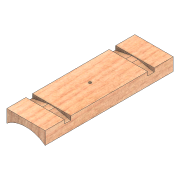
# Autodesk Inventor part: legno 2
Saved by Autodesk Inventor 2022 (Build 260153000, 153)
## iProperties
Created: 2025-08-09
Part Number: legno 2
Material: Wood (Birch)
Document SubType Name: Modeling
Designer: sacchie
Density: 0.55 g/cm^3
Appearance: Birch - Natural Polished
Author: sacchie
Autodesk Inventor part; units mm, degrees
ref_plane "YZ Plane" through (0, 0, 0) normal (1, 0, 0) x (0, 1, 0)
sketch "Sketch1" plane through (0, 0, 0) normal (0, 0, 1) x (1, 0, 0)
  line L0 (0, 0) -> (-20, 0)
  line L1 (-20, 0) -> (-20, 10)
  line L2 (-20, 10) -> (0, 10)
  line L3 (0, 10) -> (0, 0)
  line L4 (-10, 0) -> (24.641, 0) construction
  line L5 (-10, 0) -> (24.641, 0) construction
  line L6 (0, 10) -> (20, 10)
  line L7 (20, 10) -> (20, -10)
  line L8 (-20, 10) -> (-40, 10)
  line L9 (-40, 10) -> (-40, -10)
  arc A0 (20, -10) -> (-40, -10) centre (-10, -48.9954) ccw
  point P0 (-5.5176, 0)
  point P1 (-14.4824, 0)
  dimension "d0" = 20
  dimension "d1" = 10
  dimension "d8" = 30
  dimension "d10" = 30
  dimension "d15" = 20
  dimension "d16" = 20
  constraints: 20 end point, 4 horizontal, 3 perpendicular, 2 parallel, 2 point on circle, 1 centre point, 1 midpoint, 1 point on line
  measures "d0" distance of L1.end L2.end
  measures "d1" distance of L0.end L1.end
  measures "d8" horizontal distance of L9.end L4.start
  measures "d10" horizontal distance of L7.end L4.start
  measures "d15" distance of L8.end L9.end
  measures "d16" distance of L6.end L7.end
extrude "Extrusion1" add sketch "Sketch1" along normal blind 200
sketch "Sketch4" plane through (-40, 10, 0) normal (0, 1, 0) x (1, 0, 0)
  line L0 (0, 0) -> (0, -200) projected
  line L1 (60, 0) -> (60, -200) projected
  line L2 (0, 0) -> (60, -200) construction
  circle A0 centre (30, -100) radius 2
  point P0 (40, 0)
  dimension "d17" = 4
  constraints: 2 end point, 1 centre point, 1 midpoint
  measures "d17" diameter of A0
extrude "Extrusion4" cut sketch "Sketch4" against normal through all
ref_plane "Work Plane1" through (0, 0, 170) normal (0, 0, 1) x (1, 0, 0)
sketch "Sketch5" plane through (0, 0, 200) normal (0, 0, 1) x (1, 0, 0)
  line L0 (20, 10) -> (-40, 10) projected
  line L1 (-10, 10) -> (-40, 4)
  line L2 (-10, 10) -> (-40, 10)
  line L3 (-40, 4) -> (-40, 10)
  line L4 (-10, 10) -> (-10, 14.555) construction
  line L5 (-40, 10) -> (20, 10)
  line L6 (-10, 10) -> (20, 4)
  line L7 (-10, 10) -> (20, 10)
  line L8 (20, 4) -> (20, 10)
  line L9 (-15, 9) -> (-5, 9)
  point P0 (0, 0)
  dimension "d21" = 6
  dimension "d24" = 1
  constraints: 18 end point, 3 symmetric about line, 2 point on line, 1 collinear, 1 horizontal, 1 midpoint, 1 vertical
  measures "d21" distance of L1.end L0.end
  measures "d24" distance between parallel lines of L0 L9
extrude "Extrusion5" cut sketch "Sketch5" against normal blind 10 from surface at -30
ref_plane "Work Plane2" through (0, 0, 100) normal (0, 0, 1) x (1, 0, 0)
mirror "Mirror1" about plane through (0, 0, 100) normal (0, 0, 1) of "Extrusion5"
equation "\"d10\" = d8"
equation "\"d16\" = d15"
body "Solid1"
